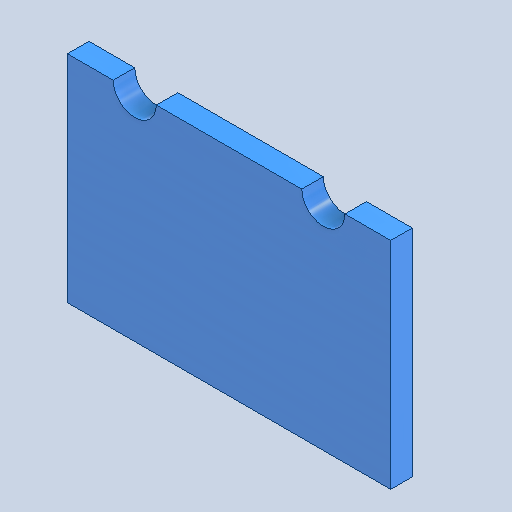
# Autodesk Inventor part: 支撑板1
Saved by Autodesk Inventor 2022 (Build 260153000, 153)
## iProperties
Created: 2023-02-22
Part Number: 支撑板1
Material: 常规
Document SubType Name: Modeling
Designer: 李承轩
Density: 1 g/cm^3
Appearance: 青色
Author: 李承轩
Autodesk Inventor part; units mm, degrees
ref_plane "YZ Plane" through (0, 0, 0) normal (1, 0, 0) x (0, 1, 0)
ref_plane "XZ Plane" through (0, 0, 0) normal (0, 1, 0) x (-1, 0, 0)
ref_plane "XY Plane" through (0, 0, 0) normal (0, 0, 1) x (1, 0, 0)
sketch "草图1" plane through (0, 0, 0) normal (0, 0, 1) x (1, 0, 0)
  line L0 (150, -100) -> (-150, -100)
  line L1 (-150, -100) -> (-150, 100)
  line L2 (-150, 100) -> (150, 100)
  line L3 (150, 100) -> (150, -100)
  line L4 (150, -100) -> (-150, 100) construction
  line L5 (-150, -100) -> (150, 100) construction
  point P0 (0, 0)
  dimension "d0" = 300
  dimension "d1" = 200
  constraints: 12 end point, 2 midpoint, 2 parallel, 1 horizontal, 1 perpendicular
  measures "d0" distance of L1.end L2.end
  measures "d1" distance of L0.end L1.end
extrude "拉伸1" add sketch "草图1" along normal mid plane 20
sketch "草图2" plane through (0, 0, 10) normal (0, 0, 1) x (1, 0, 0)
  line L0 (150, 100) -> (-150, 100) construction
  line L1 (-150, 100) -> (-150, -100) construction
  line L2 (-150, -100) -> (150, -100) construction
  line L3 (150, -100) -> (150, 100) construction
  line L4 (150, 100) -> (-150, 100) construction
  circle A0 centre (-87.5, 100) radius 20
  line L5 (0, 0) -> (0, 160.0465) construction
  circle A1 centre (87.5, 100) radius 20
  dimension "d4" = 40
  dimension "d5" = 175
  constraints: 2 centre point, 2 end point, 1 point on line, 1 symmetric about line, 1 vertical, 1 other
  measures "d4" diameter of A0
  measures "d5" distance of A1.centre A0.centre
extrude "拉伸2" cut sketch "草图2" against normal blind 20
sketch "草图3" plane through (-150, -100, 10) normal (0, -1, 0) x (1, 0, 0)
  line L0 (300, -20) -> (300, 0) construction
  line L1 (0, 0) -> (300, 0) construction
  line L2 (0, -20) -> (0, 0) construction
  line L3 (300, -20) -> (0, -20) construction
  line L4 (0, -20) -> (42.5, -20) projected
  line L5 (150, -10) -> (150, 57.6375)
  line L6 (300, -20) -> (300, 0) construction
  line L7 (300, -20) -> (257.5, -20) construction
  line L8 (0, 0) -> (300, 0) projected
  line L9 (40, 0) -> (60, 0)
  line L10 (60, 0) -> (60, -50)
  line L11 (60, -50) -> (40, -50)
  line L12 (40, -50) -> (40, 0)
  line L13 (300, -20) -> (300, 0) construction
  line L14 (300, -20) -> (257.5, -20)
  line L15 (260, 0) -> (240, 0)
  line L16 (240, 0) -> (240, -50)
  line L17 (240, -50) -> (260, -50)
  line L18 (260, -50) -> (260, 0)
  point P0 (260, 0)
  point P1 (240, 0)
  dimension "d20" = 20
  dimension "d21" = 50
  dimension "d22" = 180
  constraints: 26 end point, 5 symmetric about line, 2 parallel, 2 perpendicular, 1 horizontal, 1 point on line
  measures "d20" distance of L10.end L11.end
  measures "d21" distance of L9.end L10.end
  measures "d22" distance between parallel lines of L10 L16
extrude "拉伸4" add sketch "草图3" against normal blind 10
full round fillet "全圆角3" first side at (110, -96.6667, -30) centre faces at (96.6667, -96.6667, -40) second side at (90, -96.6667, -20)
mirror "镜像1" about plane through (0, 0, 0) normal (1, 0, 0) of "全圆角3"
sketch "草图5" plane through (-150, -90, 10) normal (0, 1, 0) x (1, 0, 0)
  arc A0 (260, 40) -> (240, 40) centre (250, 40) ccw projected
  arc A1 (60, 40) -> (40, 40) centre (50, 40) ccw projected
  point P0 (150, 10)
  constraints: 2 coincident
hole "孔2" at (100, -90, -30) at (-100, -90, -30) direction (0, -1, 0) diameter 10 end through all
